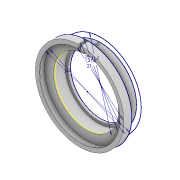
# Autodesk Inventor part: 32to25mmFilterAdapter
Saved by Autodesk Inventor 2021 (Build 250183000, 183)
## iProperties
Created: 2022-11-22
Part Number: 32to25mmFilterAdapter
Material: Generic
Document SubType Name: Modeling
Designer: nvladi
Density: 1 g/cm^3
Appearance: Default
Author: nvladi
Autodesk Inventor part; units mm, degrees
ref_plane "YZ Plane" through (0, 0, 0) normal (1, 0, 0) x (0, 1, 0)
ref_plane "XZ Plane" through (0, 0, 0) normal (0, 1, 0) x (-1, 0, 0)
ref_plane "XY Plane" through (0, 0, 0) normal (0, 0, 1) x (1, 0, 0)
sketch "Sketch1" plane through (0, 0, 0) normal (0, 0, 1) x (1, 0, 0)
  circle A0 centre (0, 0) radius 13.8
  circle A1 centre (0, 0) radius 11.5
  circle A2 centre (0, 0) radius 15.6
  circle A3 centre (0, 0) radius 12.5
  dimension "d0" = 27.6
  dimension "d1" = 23
  dimension "d2" = 31.2
  dimension "d3" = 25
  constraints: 4 centre point, 4 coincident
  measures "d0" diameter of A0
  measures "d1" diameter of A1
  measures "d2" diameter of A2
  measures "d3" diameter of A3
extrude "Extrusion1" add sketch "Sketch1" along normal blind 1 contours A3
extrude "Extrusion2" add sketch "Sketch1" along normal blind 4 contours A0
sketch "Sketch2" plane through (0, 0, 4) normal (0, 0, 1) x (1, 0, 0)
  circle A0 centre (0, 0) radius 15.6 projected
  circle A1 centre (0, 0) radius 12.5 projected
extrude "Extrusion3" add sketch "Sketch2" along normal blind 1
sketch "Sketch4" plane through (0, 0, 5) normal (0, 0, 1) x (1, 0, 0)
  circle A0 centre (0, 0) radius 16
  circle A1 centre (0, 0) radius 17
  circle A2 centre (0, 0) radius 12.5 projected
  dimension "d14" = 32
  dimension "d15" = 34
  constraints: 2 centre point, 2 coincident
  measures "d14" diameter of A0
  measures "d15" diameter of A1
extrude "Extrusion5" add sketch "Sketch4" along normal blind 0.5 contours A0
extrude "Extrusion6" add sketch "Sketch4" along normal blind 3 contours A1
sketch "Sketch5" plane through (0, 0, 8) normal (0, 0, 1) x (1, 0, 0)
  circle A0 centre (0, 0) radius 16 projected
  circle A1 centre (0, 0) radius 15.5
  dimension "d20" = 31
  constraints: 1 centre point, 1 coincident
  measures "d20" diameter of A1
extrude "Extrusion7" add sketch "Sketch5" against normal blind 0.25
sketch "Sketch8" plane through (0, 0, 8) normal (0, 0, 1) x (1, 0, 0)
  line L0 (0.5, 10) -> (-0.5, 10)
  line L1 (-0.5, 10) -> (-0.5, 20)
  line L2 (-0.5, 20) -> (0.5, 20)
  line L3 (0.5, 20) -> (0.5, 10)
  circle A0 centre (0, 0) radius 15 projected
  line L4 (0.5, 10) -> (-0.5, 20) construction
  line L5 (-0.5, 10) -> (0.5, 20) construction
  point P0 (0, 15)
  dimension "d30" = 1
  dimension "d31" = 10
  constraints: 12 end point, 2 midpoint, 2 parallel, 1 horizontal, 1 perpendicular, 1 vertical alignment, 1 other
  measures "d30" distance of L1.end L2.end
  measures "d31" distance of L0.end L1.end
extrude "Extrusion10" cut sketch "Sketch8" against normal blind 10 contours L0 L1 A0 L3 | A0 L1 L2 L3 picked at (-0.0556, 11.6664)
body "Solid1"
